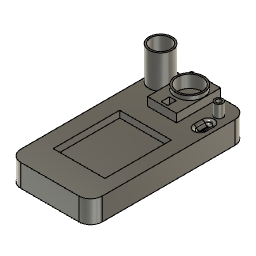
FinalLamp (Autodesk Fusion 360 archive; units mm, degrees)
design "Base"
Autodesk Fusion 360 part; units mm, degrees
sketch "Sketch1" plane through (0, 0, 0) normal (0, 0, 1) x (1, 0, 0)
  line L0 (35, 94) -> (-35, 94)
  line L1 (-49, 80) -> (-49, -80)
  line L2 (-35, -94) -> (35, -94)
  line L3 (49, -80) -> (49, 80)
  line L4 (49, 94) -> (-49, -94) construction
  line L5 (-49, 94) -> (49, -94) construction
  arc A0 (-35, 94) -> (-49, 80) centre (-35, 80) ccw
  arc A1 (49, 80) -> (35, 94) centre (35, 80) ccw
  arc A2 (-49, -80) -> (-35, -94) centre (-35, -80) ccw
  arc A3 (35, -94) -> (49, -80) centre (35, -80) ccw
  line L6 (0, 94) -> (0, 74.271) construction
  line L7 (-49, 58) -> (49, 58) construction
  circle A4 centre (0, 74.271) radius 17
  line L8 (0, 74.271) -> (-35, 74.271) construction
  circle A5 centre (-35, 74.271) radius 14
  circle A6 centre (0, 74.271) radius 15
  circle A7 centre (-35, 74.271) radius 12
  line L9 (0, 74.271) -> (35, 74.271)
  circle A8 centre (35, 74.271) radius 5
  circle A9 centre (35, 74.271) radius 3
  line L10 (-17.5, 94) -> (-17.5, 41)
  line L11 (-17.5, 41) -> (17.5, 41)
  line L12 (17.5, 41) -> (17.5, 94)
  line L13 (-4.032, 54) -> (3.968, 54)
  line L14 (3.968, 54) -> (3.968, 44)
  line L15 (3.968, 44) -> (-4.032, 44)
  line L16 (-4.032, 44) -> (-4.032, 54)
  line L17 (-30, 20) -> (32.22, 20)
  line L18 (32.22, 20) -> (32.22, -60)
  line L19 (32.22, -60) -> (-30, -60)
  line L20 (-30, -60) -> (-30, 20)
  dimension "d1" = 98
  dimension "d2" = 188
  dimension "d3" = 14
  dimension "d4" = 14
  dimension "d5" = 14
  dimension "d6" = 14
  dimension "d8" = 70
  dimension "d9" = 36
  dimension "d14" = 35
  constraint horizontal L0
  constraint perpendicular L0 L1
  constraint parallel L0 L2
  constraint parallel L1 L3
  constraint coincident L4 origin
  constraint coincident L5 origin
  constraint coincident L5.start L0
  constraint coincident L5.start L1
  constraint tangent L0 A0
  constraint tangent L1 A0
  constraint coincident L4.start L0
  constraint coincident L4.start L3
  constraint tangent L0 A1
  constraint tangent L3 A1
  constraint coincident L4.end L1
  constraint coincident L4.end L2
  constraint tangent L1 A2
  constraint tangent L2 A2
  constraint coincident L5.end L3
  constraint coincident L5.end L2
  constraint tangent L3 A3
  constraint tangent L2 A3
  constraint midpoint L0 L6.start
  constraint perpendicular L0 L6
  constraint coincident L1 L7.start
  constraint coincident L3 L7.end
  constraint perpendicular L3 L7
  constraint coincident L6.end A4.centre
  constraint perpendicular L6 L8
  constraint coincident L8.end A5.centre
  constraint concentric A4 A6
  constraint concentric A5 A7
  constraint perpendicular L6 L9
  constraint coincident L9.end A8.centre
  constraint concentric A8 A9
  constraint coincident L0 L10.start
  constraint perpendicular L0 L10
  constraint perpendicular L10 L11
  constraint coincident L0 L12.end
  constraint perpendicular L0 L12
  constraint horizontal L13
  constraint vertical L14
  constraint horizontal L15
  constraint vertical L16
  constraint horizontal L17
  constraint vertical L18
  constraint horizontal L19
  constraint vertical L20
  measures "d1" distance of L4.end L5.end
  measures "d2" distance of L5.start L4.end
  measures "d3" radius of A0
  measures "d4" radius of A1
  measures "d5" radius of A2
  measures "d6" radius of A3
  measures "d8" distance of L0.end L0.start
  measures "d9" distance of L0 L7
  measures "d14" distance of L6.end L9.end
extrude "Extrude1" add sketch "Sketch1" along normal blind 40 contours A5 makes body 1
extrude "Extrude2" add sketch "Sketch1" along normal blind 10 separate body contours L0 L10 L11 L12 makes body 2
extrude "Extrude3" add sketch "Sketch1" along normal blind 15 contours A4 bodies 2
extrude "Extrude4" add sketch "Sketch1" along normal blind 15 separate body contours A8 makes body 3
surface "Extrude5" add extruded along (0, 0, 1) between 0 and -8 profiles "Sketch1" section 1 contours L17 L18 L19 L20 separate body makes body 4
sketch "Sketch2" plane through (0, 0, 0) normal (0, 0, 1) x (1, 0, 0)
  line L0 (-30, -60) -> (32.22, -60)
  line L1 (32.22, -60) -> (32.22, 20)
  line L2 (32.22, 20) -> (-30, 20)
  line L3 (-30, 20) -> (-30, -60)
  constraint horizontal L0
  constraint vertical L1
  constraint horizontal L2
  constraint vertical L3
extrude "Extrude6" add sketch "Sketch1" against normal blind 27 separate body contours L0 L1 L2 L3 A0 A1 A2 A3 L10 L11 L12 | L17 L18 L19 L20 makes body 5
extrude "Extrude7" cut sketch "Sketch2" against normal blind 8 bodies 5
extrude "Extrude8" add sketch "Sketch1" against normal blind 27 contours L0 L10 L11 L12 bodies 2 5
extrude "Extrude9" add sketch "Sketch1" against normal blind 27 separate body contours A6 makes body 6
extrude "Extrude10" add sketch "Sketch1" against normal blind 27 separate body contours L13 L14 L15 L16 makes body 7
extrude "Extrude11" add sketch "Sketch1" against normal blind 27 separate body contours A7 makes body 8
extrude "Extrude12" add sketch "Sketch1" against normal blind 27 separate body contours A9 makes body 9
extrude "Extrude13" add 1 faces at (-21.7635, 72.9793, 0) along direction (0, 0, -1) blind 27 on bodies 1 bodies 1 3 6 7 9 2 8
extrude "Extrude14" add 1 faces at (16.27, 73.4264, 0) along direction (0, 0, -1) blind 27 on bodies 1 bodies 1 6
extrude "Extrude15" add 1 faces at (30.6853, 74.5194, 0) along direction (0, 0, -1) blind 27 on bodies 3 bodies 3 7 1 9
sketch "Sketch3" plane through (0, 0, 0) normal (0, 0, 1) x (-1, 0, 0)
  line L0 (-32.22, 60) -> (30, 60)
  line L1 (30, 60) -> (30, -20)
  line L2 (30, -20) -> (-32.22, -20)
  line L3 (-32.22, -20) -> (-32.22, 60)
  circle A0 centre (-35, -74.271) radius 5
  line L4 (17.5, -94) -> (35, -94)
  arc A1 (35, -94) -> (49, -80) centre (35, -80) ccw
  line L5 (49, -80) -> (49, -74.271)
  circle A2 centre (35, -74.271) radius 14
  line L6 (49, -74.271) -> (49, 80)
  arc A3 (49, 80) -> (35, 94) centre (35, 80) ccw
  line L7 (35, 94) -> (-35, 94)
  arc A4 (-35, 94) -> (-49, 80) centre (-35, 80) ccw
  line L8 (-49, 80) -> (-49, -80)
  arc A5 (-49, -80) -> (-35, -94) centre (-35, -80) ccw
  line L9 (-35, -94) -> (-17.5, -94)
  line L10 (-17.5, -94) -> (-17.5, -41)
  line L11 (-17.5, -41) -> (17.5, -41)
  line L12 (17.5, -41) -> (17.5, -94)
  line L13 (-33, -60) -> (-33, -50)
  line L14 (-40, -60) -> (-40, -50)
  arc A6 (-33, -50) -> (-40, -50) centre (-36.5, -50) ccw
  arc A7 (-40, -60) -> (-33, -60) centre (-36.5, -60) ccw
  constraint parallel L8 L13
  constraint perpendicular L11 L14
  constraint tangent L13 A6
  constraint tangent L14 A6
  constraint tangent L13 A7
extrude "Extrude16" cut sketch "Sketch3" against normal blind 4 contours L13 L14 A6 A7 bodies 3
fillet "Fillet1" radius 4 4 edges at (36.5, 63.5, 0) (40, 55, 0) (36.5, 46.5, 0) (33, 55, 0) 1 faces at (37.6667, 53.3333, -4) on bodies 3
component "Component" placed x (1, 0, 0) y (0, 1, 0) z (0, 0, 1) at (0, 0, 0)

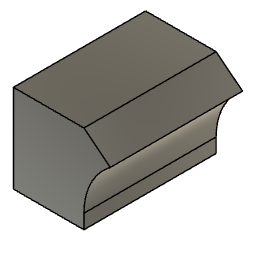
design "Switch"
Autodesk Fusion 360 part; units mm, degrees
sketch "Sketch1" plane through (0, 0, 0) normal (0, 1, 0) x (1, 0, 0)
  line L0 (0, 0) -> (8, 0)
  line L1 (8, 0) -> (8, -10)
  line L2 (8, -10) -> (0, -10)
  line L3 (0, -10) -> (0, 0)
  line L4 (8, -10) -> (10.9985, -7.6243)
  arc A0 (8.1775, -0.0036) -> (8, 0) centre (8, -4.4018) ccw construction
  arc A1 (8.1775, -0.0036) -> (10.9985, -7.6243) centre (15.5, -1.6254) ccw
  constraint horizontal L0
  constraint vertical L1
  constraint horizontal L2
  constraint vertical L3
  constraint coincident L0.start L3.end
  constraint tangent L1 A1
  constraint tangent L0 A0
extrude "Extrude1" add sketch "Sketch1" along normal blind 15

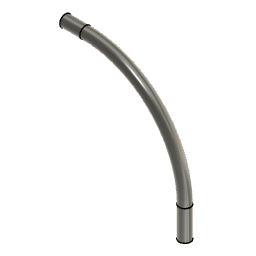
design "Pipefinal"
Autodesk Fusion 360 part; units mm, degrees
sketch "Sketch1" plane through (0, 0, 0) normal (0, 1, 0) x (1, 0, 0)
  line L0 (61.566, 226.2366) -> (61.566, 147.3725)
  line L1 (-251.8441, -113.4675) -> (-199.274, -113.4675)
  arc A0 (-199.274, -113.4675) -> (61.566, 147.3725) centre (-199.274, 147.3725) ccw
  point P0 (61.566, 157.6566)
  point P1 (-201.8441, -113.4675)
  constraint vertical L0
  constraint horizontal L1
  constraint coincident P1 L1
  constraint coincident P0 L0
  constraint tangent L1 A0
  constraint tangent L0 A0
pipe "Pipe1" add diameter 30 wall 2 path "Sketch1" along L0 A0 L1

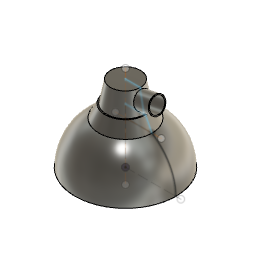
design "Lamp"
Autodesk Fusion 360 part; units mm, degrees
sketch "Sketch1" plane through (0, 0, 0) normal (0, 1, 0) x (1, 0, 0)
  line L0 (0, -110) -> (0, 0) construction
  line L1 (0, 0) -> (110, 0) construction
  arc A0 (48.775, -85) -> (98, 0) centre (0, 0) ccw
  arc A1 (52.6783, -85) -> (100, 0) centre (0, 0) ccw
  spline S0 degree 5 poles (-20.0054, -85) (-16.3635, -85) (-9.0799, -85) (1.8456, -85) (16.4129, -85) (34.6221, -85) (49.1894, -85) (60.1149, -85) (67.3986, -85) (71.0404, -85) knots 0 0 0 0 0 0 0.2 0.4 0.6 0.8 1 1 1 1 1 1
  line L2 (0, -85) -> (52.6783, -85)
  line L3 (0, -110) -> (40, -110)
  line L4 (40, -110) -> (52.6783, -85)
  line L5 (0, -108) -> (38.7718, -108)
  line L6 (38.7718, -108) -> (50.8945, -84.0954)
  line L7 (0, -151.9119) -> (29.6292, -151.9119)
  line L8 (29.6292, -151.9119) -> (37.7575, -110)
  line L9 (0, -170) -> (0, 30) construction
  line L10 (98, 0) -> (100, 0)
  line L11 (0, -110) -> (0, -108)
  line L12 (0, -151.9119) -> (0, -149.9119)
  line L13 (0, -149.9119) -> (27.9798, -149.9119)
  line L14 (27.9798, -149.9119) -> (35.7941, -109.6192)
  dimension "d3" = 85
  dimension "d4" = 100
  dimension "d5" = 98
  dimension "d6" = -2
  dimension "d7" = -2
  constraint coincident L0.end L1.start
  constraint vertical L0
  constraint perpendicular L0 L1
  constraint coincident L1 A0.end
  constraint coincident L1 A1.end
  constraint coincident S0 A1.start
  constraint coincident S0 A0.start
  constraint coincident S0 L2.start
  constraint coincident L0 L2.start
  constraint perpendicular L0 L2
  constraint perpendicular L0 L3
  constraint horizontal L7
  constraint coincident L3 L8.end
  constraint perpendicular L1 L9
  measures "d3" distance of L1 L2
  measures "d4" radius of A1
  measures "d5" radius of A0
revolve "Revolve1" add sketch "Sketch1" angle 360 about axis through (0, 0, 170) along (0, 0, -1) contours S0 L2 L3 L4 L5 L6 L11
revolve "Revolve2" add sketch "Sketch1" angle 360 about axis through (0, 0, 170) along (0, 0, -1) contours A0 A1 S0 L2 L10
sketch "Sketch2" plane through (0, 0, 0) normal (0, 1, 0) x (1, 0, 0)
revolve "Revolve3" add sketch "Sketch1" angle 360 about axis through (0, 0, 170) along (0, 0, -1) contours L3 L7 L8 L12 L13 L14
sketch "Sketch3" plane through (0, 0, 0) normal (0, 1, 0) x (1, 0, 0)
  line L0 (30, -149) -> (33.3885, -132.3411)
  line L1 (30, -149) -> (59.398, -154.9797)
  line L2 (33.3885, -132.3411) -> (62.7865, -138.3208)
  line L3 (33.3885, -132.3411) -> (88.2617, -143.5025) construction
  line L4 (32.3585, -147.4388) -> (59.7967, -153.0198)
  line L5 (59.398, -154.9797) -> (59.7967, -153.0198)
  line L6 (32.3585, -147.4388) -> (30.3986, -147.0401)
  dimension "d13" = 30
  constraint perpendicular L0 L1
  constraint perpendicular L0 L3
  constraint parallel L1 L4
  constraint perpendicular L1 L5
  constraint coincident L0 L6.end
  constraint perpendicular L0 L6
  measures "d13" distance of L0.start L1.end
revolve "Revolve4" add sketch "Sketch3" angle 360 about axis through (33.3885, 0, 132.3411) along (0.979934, 0, 0.199322)
